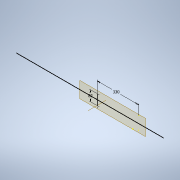
# Autodesk Inventor part: union_frenos
Saved by Autodesk Inventor 2021 (Build 250183000, 183)
## iProperties
Created: 2021-07-10
Part Number: union_frenos
Material: Generic
Document SubType Name: Modeling
Designer: j2seb
Density: 1 g/cm^3
Appearance: Default
Author: j2seb
Autodesk Inventor part; units mm, degrees
ref_plane "YZ Plane" through (0, 0, 0) normal (1, 0, 0) x (0, 1, 0)
ref_plane "XZ Plane" through (0, 0, 0) normal (0, 1, 0) x (-1, 0, 0)
ref_plane "XY Plane" through (0, 0, 0) normal (0, 0, 1) x (1, 0, 0)
ref_plane "Work Plane1" through (-1250.62, 0, 0) normal (0, 0, 1) x (1, 0, 0)
sketch "Sketch1" plane through (-1250.62, 0, 0) normal (0, 0, 1) x (1, 0, 0)
  line L0 (334.6073, 62.526) -> (1495.298, 62.526)
  line L1 (1300.7701, 117.526) -> (1295.7701, 117.526) projected
  line L2 (1295.7701, 17.526) -> (1300.7701, 17.526) projected
  line L3 (1050.7701, 21.526) -> (1050.7701, 103.526)
  point P0 (1250.62, 0)
  point P1 (1050.7701, 62.526)
  dimension "d0" = 82
  dimension "d1" = 250
  constraints: 4 end point, 2 coincident, 1 horizontal, 1 horizontal alignment, 1 midpoint, 1 vertical, 2 other
  measures "d0" distance of L3.start L3.end
  measures "d1" distance from line of L1.start L3
sketch "Sketch2" plane through (-1250.62, 0, 0) normal (0, 0, 1) x (1, 0, 0)
  circle A0 centre (1050.7701, 21.526) radius 5
  circle A1 centre (1050.7701, 103.526) radius 5
  point P0 (1250.62, 0)
  dimension "d2" = 10
  dimension "d3" = 10
  constraints: 2 centre point, 2 coincident
  measures "d2" diameter of A0
  measures "d3" diameter of A1
extrude "Extrusion1" add sketch "Sketch2" against normal blind 5
body "Solid1"
